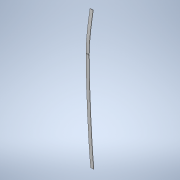
# Autodesk Inventor part: cowl_insulation
Saved by Autodesk Inventor 2020.3 (Build 243373010, 373A)
## iProperties
Created: 2021-01-30
Part Number: cowl_insulation
Material: Generic
Document SubType Name: Modeling
Designer: kardo
Density: 1 g/cm^3
Appearance: Default
Author: kardo
Autodesk Inventor part; units mm, degrees
ref_plane "YZ Plane" through (0, 0, 0) normal (1, 0, 0) x (0, 1, 0)
ref_plane "XZ Plane" through (0, 0, 0) normal (0, 1, 0) x (-1, 0, 0)
ref_plane "XY Plane" through (0, 0, 0) normal (0, 0, 1) x (1, 0, 0)
derived "cowl_strip.ipt"
sketch "Sketch10" plane through (-19.176, -306, 32.793) normal (1, 0, 0) x (0, 1, 0)
  line L0 (306, 14.025) -> (308, 14.025)
  line L1 (306, 12.825) -> (308, 12.825)
  line L2 (0, 0) -> (0.1095, -1.195)
  line L3 (418.2, 1.8222) -> (417.9951, 0.6398)
  spline S0 degree 4 poles (0, 0) (76.3997, 6.9994) (152.9397, 9.8189) (229.4355, 14.025) (306, 14.025) knots 0 0 0 0 0 1 1 1 1 1
  spline S1 degree 3 poles (308, 14.025) (344.6041, 14.025) (380.6024, 8.3365) (418.2, 1.8222) knots 0 0 0 0 1 1 1 1
  spline S2 degree 3 poles (0.1095, -1.195) (8.5929, -0.4178) (25.5649, 1.021) (46.79, 2.5896) (68.0212, 4.0216) (85.0104, 5.0701) (106.2508, 6.2831) (123.2458, 7.1829) (144.4919, 8.231) (161.4903, 9.0108) (182.7395, 9.9118) (199.7397, 10.5713) (220.9905, 11.3066) (237.9916, 11.8164) (259.2434, 12.3313) (280.4957, 12.7085) (297.4983, 12.825) (306, 12.825) knots 0 0 0 0 0.083333 0.166667 0.208333 0.291667 0.333333 0.416667 0.458333 0.541667 0.583333 0.666667 0.708333 0.791667 0.833333 0.916667 1 1 1 1
  spline S3 degree 3 poles (308, 12.825) (311.04, 12.825) (317.1122, 12.7463) (324.6897, 12.4649) (332.2623, 12.0569) (338.3186, 11.6332) (345.8914, 10.9926) (351.9536, 10.3955) (359.5409, 9.5537) (365.6205, 8.8082) (373.2368, 7.7968) (379.3453, 6.9281) (388.5368, 5.5485) (400.8484, 3.584) (411.7307, 1.7252) (417.9951, 0.6398) knots 0 0 0 0 0.083333 0.166667 0.208333 0.291667 0.333333 0.416667 0.458333 0.541667 0.583333 0.666667 0.708333 0.833333 1 1 1 1
  point P0 (362.1, 10.4429)
  point P1 (204, 11.9136)
  point P2 (102, 7.2364)
derived "base_sketch.ipt"
extrude "Extrusion1" add sketch "Sketch10" along normal blind 9
equation "\"d2\" = cowl_insulation_width + 0.5 * cowl_strip_width"
equation "\"cowl_insulation_width\" = 6"
equation "\"cowl_strip_width\" = 6"
body "Solid1"
